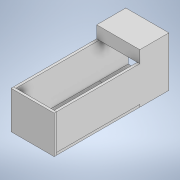
# Autodesk Inventor part: charger2
Saved by Autodesk Inventor 2020 (Build 240168000, 168)
## iProperties
Created: 2021-04-03
Part Number: charger2
Material: Generic
Document SubType Name: Modeling
Designer: Vlasciar
Density: 1 g/cm^3
Appearance: Default
Author: Vlasciar
Autodesk Inventor part; units mm, degrees
ref_plane "YZ Plane" through (0, 0, 0) normal (1, 0, 0) x (0, 1, 0)
ref_plane "XZ Plane" through (0, 0, 0) normal (0, 1, 0) x (-1, 0, 0)
ref_plane "XY Plane" through (0, 0, 0) normal (0, 0, 1) x (1, 0, 0)
sketch "Sketch1" plane through (0, 0, 0) normal (0, 1, 0) x (-1, 0, 0)
  line L0 (-8.875, -23.125) -> (8.875, -23.125)
  line L1 (8.875, -23.125) -> (8.875, 23.125)
  line L2 (8.875, 23.125) -> (-8.875, 23.125)
  line L3 (-8.875, 23.125) -> (-8.875, -23.125)
  line L4 (-8.875, -23.125) -> (8.875, 23.125) construction
  line L5 (8.875, -23.125) -> (-8.875, 23.125) construction
  point P0 (0, 0)
  dimension "d0" = 17.75
  dimension "d1" = 46.25
  constraints: 12 end point, 2 midpoint, 2 parallel, 1 horizontal, 1 perpendicular
  measures "d0" distance between parallel lines of L3 L1
  measures "d1" distance between parallel lines of L0 L2
extrude "Extrusion1" add sketch "Sketch1" along normal blind 20.5
sketch "Sketch2" plane through (0, 20.5, 0) normal (0, 1, 0) x (1, 0, 0)
  line L0 (-8.875, 23.125) -> (-8.875, -23.125) projected
  line L1 (-8.875, -23.125) -> (8.875, -23.125) projected
  line L2 (8.875, -23.125) -> (8.875, 23.125) projected
  line L3 (8.875, 23.125) -> (-8.875, 23.125) projected
  line L4 (-8.875, 11.125) -> (8.875, 11.125)
  point P0 (0, 0)
  dimension "d4" = 12
  constraints: 2 end point, 2 point on line, 1 perpendicular
  measures "d4" distance between parallel lines of L3 L4
extrude "Extrusion2" cut sketch "Sketch2" against normal blind 5 contours L4 L2 L1 L0
shell "Shell1" thickness 1 removed faces 1 at (-2.9583, 15.5, 0.2917)
shell "Shell2" thickness 1 removed faces 2 at (2.9583, 13.6667, -23.125) at (2.625, 13.3333, -22.125)
sketch "Sketch3" plane through (-8.875, 0, 23.125) normal (0, 0, 1) x (1, 0, 0)
  line L0 (17.75, 0) -> (17.75, 15.5) projected
  line L1 (0, 7) -> (18, 7)
  line L2 (1, 15.5) -> (16.75, 15.5) projected
  line L3 (8.875, 15.5) -> (8.875, 0)
  point P0 (8.875, 7)
  constraints: 4 end point, 2 perpendicular, 2 point on line, 1 midpoint
hole "Hole1" at (0, 7, 23.125) direction (0, 0, -1) diameter 7 depth 8 tip angle 118
sketch "Sketch4" plane through (0, 0, 0) normal (0, -1, 0) x (1, 0, 0)
  circle A0 centre (0, -13.599) radius 3
  point P0 (0, 0)
  dimension "d16" = 6
  constraints: 1 centre point
  measures "d16" diameter of A0
extrude "Extrusion3" add sketch "Sketch4" along normal blind 3.5
sketch "Sketch5" plane through (0, -3.5, -13.599) normal (0, -1, 0) x (1, 0, 0)
  circle A0 centre (0, 0) radius 3 projected
  circle A1 centre (0, 0) radius 4.5
  point P0 (0, 13.599)
  dimension "d19" = 9
  constraints: 1 centre point, 1 coincident
  measures "d19" diameter of A1
extrude "Extrusion4" add sketch "Sketch5" along normal blind 2 contours A0 | A1
sketch "Sketch6" plane through (0, -5.5, -13.599) normal (0, -1, 0) x (1, 0, 0)
  circle A0 centre (0, 0) radius 4.5 projected
  line L0 (-3, -4.5) -> (3, -4.5)
  line L1 (3, -4.5) -> (3, 4.5)
  line L2 (3, 4.5) -> (-3, 4.5)
  line L3 (-3, 4.5) -> (-3, -4.5)
  line L4 (-3, -4.5) -> (3, 4.5) construction
  line L5 (3, -4.5) -> (-3, 4.5) construction
  point P0 (0, 13.599)
  point P1 (3, 3.3541)
  point P2 (3, -3.3541)
  point P3 (-3, -3.3541)
  point P4 (-3, 3.3541)
  dimension "d22" = 6
  constraints: 12 end point, 2 midpoint, 2 parallel, 1 horizontal, 1 perpendicular
  measures "d22" distance of L2.end L1.end
extrude "Extrusion5" cut sketch "Sketch6" against normal blind 2 contours A0 L1 | L3 A0
sketch "Sketch7" plane through (7.875, 15.5, 22.125) normal (0, 0, -1) x (-1, 0, 0)
  circle A0 centre (7.875, -8.5) radius 3.5 projected
  line L0 (0, 0) -> (15.75, 0) projected
  line L1 (0, -14.5) -> (0, 0) projected
  line L2 (15.75, -14.5) -> (0, -14.5) projected
  line L3 (15.75, -14.5) -> (15.75, 0) projected
  point P0 (7.875, -15.5)
extrude "Extrusion6" cut sketch "Sketch7" against normal blind 2
sketch "Sketch8" plane through (-7.875, 1, 23.125) normal (0, 1, 0) x (1, 0, 0)
  line L0 (15.75, 0) -> (0, 0) projected
  line L1 (0, 34.25) -> (0, 35.25) projected
  line L2 (-1, 46.25) -> (-1, 0) projected
  line L3 (16.75, -1) -> (-1, -1)
  line L4 (-1, -1) -> (-1, 34.25)
  line L5 (-1, 34.25) -> (16.75, 34.25)
  line L6 (16.75, 34.25) -> (16.75, -1)
  point P0 (7.875, 23.125)
  dimension "d27" = 1
  constraints: 8 end point, 2 parallel, 1 horizontal, 1 perpendicular, 1 point on line
  measures "d27" distance between parallel lines of L3 L0
extrude "Extrusion7" add sketch "Sketch8" along normal blind 1 separate body
sketch "Sketch9" plane through (-7.875, 2, 23.125) normal (0, 1, 0) x (1, 0, 0)
  line L0 (16.75, -1) -> (16.75, 34.25) projected
  line L1 (-1, 34.25) -> (-1, -1) projected
  line L2 (-1, -1) -> (16.75, -1) projected
  line L3 (16.75, -1) -> (-1, -1)
  line L4 (-1, -1) -> (-1, 0)
  line L5 (-1, 0) -> (16.75, 0)
  line L6 (16.75, 0) -> (16.75, -1)
  point P0 (7.875, 23.125)
  point P1 (-1, 0)
  constraints: 8 end point, 2 parallel, 1 horizontal, 1 perpendicular
extrude "Extrusion8" add sketch "Sketch9" along normal blind 15 bodies 2
move or copy body "Move Body1" bodies to move or copy 2 copy no translate (0, -1, 0)
sketch "Sketch10" plane through (-8.875, 16, 24.125) normal (0, 1, 0) x (1, 0, 0)
  line L0 (0, 0) -> (17.75, 0) projected
  line L1 (17.75, 0) -> (17.75, 1) projected
  line L2 (17.75, 1) -> (0, 1) projected
  line L3 (0, 1) -> (0, 0) projected
  point P0 (8.875, 24.125)
extrude "Extrusion9" cut sketch "Sketch10" against normal blind 0.5 bodies 2
body "Solid1"
body "Solid2"
